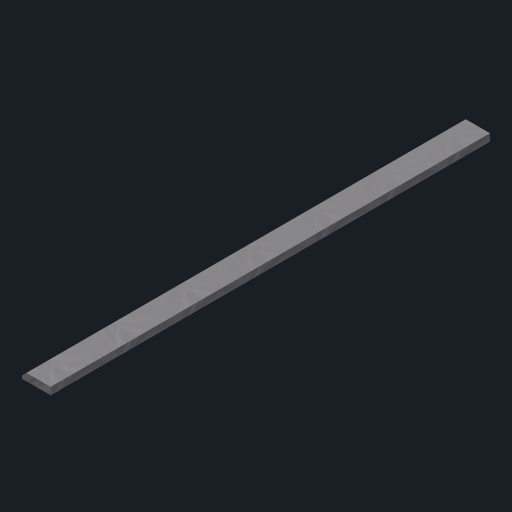
# Autodesk Inventor part: SEPARADOR
Saved by Autodesk Inventor 2024.3 (Build 283343000, 343)
## iProperties
Created: 2024-07-03
Part Number: SEPARADOR
Material: Steel, Mild, Welded
Document SubType Name: Modeling
Designer: Niler
Density: 7.85 g/cm^3
Appearance: Weld - Steel Mild
Author: Niler
Autodesk Inventor part; units mm, degrees
ref_plane "YZ Plane" through (0, 0, 0) normal (1, 0, 0) x (0, 1, 0)
ref_plane "XZ Plane" through (0, 0, 0) normal (0, 1, 0) x (-1, 0, 0)
ref_plane "XY Plane" through (0, 0, 0) normal (0, 0, 1) x (1, 0, 0)
sketch "Sketch1" plane through (0, 0, 0) normal (0, 1, 0) x (-1, 0, 0)
  line L0 (-9.75, 149.5) -> (9.75, 149.5)
  line L1 (9.75, 149.5) -> (9.75, -149.5)
  line L2 (9.75, -149.5) -> (-9.75, -149.5)
  line L3 (-9.75, -149.5) -> (-9.75, 149.5)
  line L4 (-9.75, 149.5) -> (9.75, -149.5) construction
  line L5 (9.75, 149.5) -> (-9.75, -149.5) construction
  point P0 (0, 0)
  dimension "d0" = 19.5
  dimension "d1" = 299
  constraints: 12 end point, 2 midpoint, 2 parallel, 1 horizontal, 1 perpendicular
  measures "d0" distance of L1.end L2.end
  measures "d1" distance of L0.end L1.end
extrude "Extrusion1" add sketch "Sketch1" along normal blind 5
chamfer "Chamfer1" distance 3 angle 45 1 edges at (-9.75, 5, 0)
body "Solid1"
